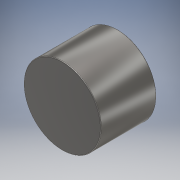
# Autodesk Inventor part: LoadTestBlock
Saved by Autodesk Inventor 2018 (Build 220112000, 112)
## iProperties
Created: 2017-10-24
Part Number: LoadTestBlock
Material: Steel, Carbon
Document SubType Name: Modeling
Designer: P136265
Density: 7.85 g/cm^3
Appearance: Semi-Polished
Mass: 69349.9 g
Surface Area: 2381.94 cm^2
Volume: 8834.39 cm^3
Author: P136265
Autodesk Inventor part; units mm, degrees
ref_plane "YZ Plane" through (0, 0, 0) normal (1, 0, 0) x (0, 1, 0)
ref_plane "XZ Plane" through (0, 0, 0) normal (0, 1, 0) x (-1, 0, 0)
ref_plane "XY Plane" through (0, 0, 0) normal (0, 0, 1) x (1, 0, 0)
sketch "Sketch1" plane through (0, 0, 0) normal (0, 1, 0) x (-1, 0, 0)
  circle A0 centre (0, 0) radius 125
  dimension "d0" = 250
  constraints: 1 centre point, 1 coincident
  measures "d0" diameter of A0
extrude "Extrusion1" add sketch "Sketch1" along normal blind 180
fillet "Fillet1" radius 2 2 edges at (125, 180, 0) (125, 0, 0)
body "Solid1"
